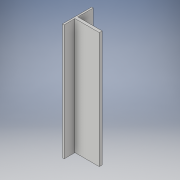
# Autodesk Inventor part: Guide 2
Saved by Autodesk Inventor 2019 (Build 230136000, 136)
## iProperties
Created: 2020-10-31
Part Number: Guide 2
Material: Generic
Document SubType Name: Modeling
Designer: Delta
Density: 1 g/cm^3
Appearance: Default
Author: Delta
Autodesk Inventor part; units mm, degrees
ref_plane "YZ Plane" through (0, 0, 0) normal (1, 0, 0) x (0, 1, 0)
ref_plane "XZ Plane" through (0, 0, 0) normal (0, 1, 0) x (-1, 0, 0)
ref_plane "XY Plane" through (0, 0, 0) normal (0, 0, 1) x (1, 0, 0)
sketch "Sketch1" plane through (0, 0, 0) normal (0, 0, 1) x (1, 0, 0)
  line L0 (0, 0) -> (3.2004, 0)
  line L1 (3.2004, 0) -> (3.2004, 228.6)
  line L2 (3.2004, 228.6) -> (0, 228.6)
  line L3 (0, 228.6) -> (0, 0)
  dimension "d0" = 3.2004
  dimension "d1" = 228.6
  constraints: 8 end point, 2 parallel, 1 horizontal, 1 perpendicular
  measures "d0" distance of L1.end L2.end
  measures "d1" distance of L0.end L1.end
extrude "Extrusion1" add sketch "Sketch1" along normal blind 57.404
sketch "Sketch2" plane through (3.2004, 0, 0) normal (1, 0, 0) x (0, 0, -1)
  line L0 (0, 0) -> (-57.404, 0) projected
  line L1 (0, 228.6) -> (-57.404, 228.6) projected
  line L2 (-35.9664, 0) -> (-30.3276, 0)
  line L3 (-30.3276, 0) -> (-30.3276, 228.6)
  line L4 (-30.3276, 228.6) -> (-35.9664, 228.6)
  line L5 (-35.9664, 228.6) -> (-35.9664, 0)
  line L6 (-57.404, 0) -> (-57.404, 228.6) projected
  dimension "d4" = 228.6
  dimension "d5" = 5.6388
  dimension "d6" = 21.4376
  constraints: 8 end point, 2 parallel, 2 point on line, 1 horizontal, 1 perpendicular
  measures "d4" distance of L2.end L3.end
  measures "d5" distance between parallel lines of L3 L5
  measures "d6" distance between parallel lines of L5 L6
extrude "Extrusion2" add sketch "Sketch2" along normal blind 47.879 contours L0 L5 L1 L3
body "Solid1"
